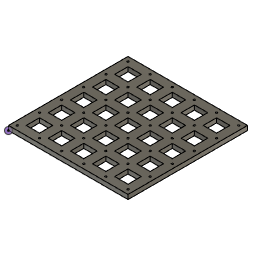
Base1 (Autodesk Fusion 360 design; units mm, degrees)
Autodesk Fusion 360 part; units mm, degrees
sketch "Sketch1" plane through (0, 0, 0) normal (0, 0, 1) x (1, 0, 0) in component "Base"
sketch "Sketch2" plane through (0, 0, 0) normal (0, 0, 1) x (1, 0, 0) in component "Base"
  line L0 (0, 0) -> (135, 0)
  line L1 (135, 0) -> (135, 135)
  line L2 (135, 135) -> (0, 135)
  line L3 (0, 135) -> (0, 0)
  line L4 (10, 10) -> (25, 10)
  line L5 (25, 10) -> (25, 25)
  line L6 (25, 25) -> (10, 25)
  line L7 (10, 25) -> (10, 10)
  line L8 (10, 35) -> (10, 50)
  line L9 (10, 50) -> (25, 50)
  line L10 (25, 50) -> (25, 35)
  line L11 (25, 35) -> (10, 35)
  line L12 (10, 60) -> (10, 75)
  line L13 (10, 75) -> (25, 75)
  line L14 (25, 75) -> (25, 60)
  line L15 (25, 60) -> (10, 60)
  line L16 (10, 85) -> (10, 100)
  line L17 (10, 100) -> (25, 100)
  line L18 (25, 100) -> (25, 85)
  line L19 (25, 85) -> (10, 85)
  line L20 (10, 110) -> (10, 125)
  line L21 (10, 125) -> (25, 125)
  line L22 (25, 125) -> (25, 110)
  line L23 (25, 110) -> (10, 110)
  line L24 (35, 125) -> (50, 125)
  line L25 (50, 125) -> (50, 110)
  line L26 (50, 110) -> (35, 110)
  line L27 (35, 110) -> (35, 125)
  line L28 (60, 110) -> (75, 110)
  line L29 (75, 110) -> (75, 125)
  line L30 (75, 125) -> (60, 125)
  line L31 (60, 125) -> (60, 110)
  line L32 (85, 110) -> (100, 110)
  line L33 (100, 110) -> (100, 125)
  line L34 (100, 125) -> (85, 125)
  line L35 (85, 125) -> (85, 110)
  line L36 (110, 110) -> (125, 110)
  line L37 (125, 110) -> (125, 125)
  line L38 (125, 125) -> (110, 125)
  line L39 (110, 125) -> (110, 110)
  line L40 (125, 100) -> (110, 100)
  line L41 (110, 100) -> (110, 85)
  line L42 (110, 85) -> (125, 85)
  line L43 (125, 85) -> (125, 100)
  line L44 (125, 75) -> (110, 75)
  line L45 (110, 75) -> (110, 60)
  line L46 (110, 60) -> (125, 60)
  line L47 (125, 60) -> (125, 75)
  line L48 (125, 50) -> (110, 50)
  line L49 (110, 50) -> (110, 35)
  line L50 (110, 35) -> (125, 35)
  line L51 (125, 35) -> (125, 50)
  line L52 (125, 25) -> (110, 25)
  line L53 (110, 25) -> (110, 10)
  line L54 (110, 10) -> (125, 10)
  line L55 (125, 10) -> (125, 25)
  line L56 (100, 10) -> (85, 10)
  line L57 (85, 10) -> (85, 25)
  line L58 (85, 25) -> (100, 25)
  line L59 (100, 25) -> (100, 10)
  line L60 (75, 10) -> (60, 10)
  line L61 (60, 10) -> (60, 25)
  line L62 (60, 25) -> (75, 25)
  line L63 (75, 25) -> (75, 10)
  line L64 (50, 10) -> (35, 10)
  line L65 (35, 10) -> (35, 25)
  line L66 (35, 25) -> (50, 25)
  line L67 (50, 25) -> (50, 10)
  line L68 (35, 35) -> (50, 35)
  line L69 (50, 35) -> (50, 50)
  line L70 (50, 50) -> (35, 50)
  line L71 (35, 50) -> (35, 35)
  line L72 (35, 60) -> (50, 60)
  line L73 (50, 60) -> (50, 75)
  line L74 (50, 75) -> (35, 75)
  line L75 (35, 75) -> (35, 60)
  line L76 (35, 85) -> (50, 85)
  line L77 (50, 85) -> (50, 100)
  line L78 (50, 100) -> (35, 100)
  line L79 (35, 100) -> (35, 85)
  line L80 (60, 100) -> (75, 100)
  line L81 (75, 100) -> (75, 85)
  line L82 (75, 85) -> (60, 85)
  line L83 (60, 85) -> (60, 100)
  line L84 (85, 100) -> (100, 100)
  line L85 (100, 100) -> (100, 85)
  line L86 (100, 85) -> (85, 85)
  line L87 (85, 85) -> (85, 100)
  line L88 (85, 75) -> (100, 75)
  line L89 (100, 75) -> (100, 60)
  line L90 (100, 60) -> (85, 60)
  line L91 (85, 60) -> (85, 75)
  line L92 (85, 50) -> (100, 50)
  line L93 (100, 50) -> (100, 35)
  line L94 (100, 35) -> (85, 35)
  line L95 (85, 35) -> (85, 50)
  line L96 (75, 35) -> (60, 35)
  line L97 (60, 35) -> (60, 50)
  line L98 (60, 50) -> (75, 50)
  line L99 (75, 50) -> (75, 35)
  line L100 (60, 60) -> (75, 60)
  line L101 (75, 60) -> (75, 75)
  line L102 (75, 75) -> (60, 75)
  line L103 (60, 75) -> (60, 60)
  circle A0 centre (5, 130) radius 1
  circle A1 centre (30, 130) radius 1
  circle A2 centre (55, 130) radius 1
  circle A3 centre (80, 130) radius 1
  circle A4 centre (105, 130) radius 1
  circle A5 centre (130, 130) radius 1
  circle A6 centre (105, 105) radius 1
  circle A7 centre (130, 105) radius 1
  circle A8 centre (5, 105) radius 1
  circle A9 centre (55, 105) radius 1
  circle A10 centre (80, 105) radius 1
  circle A11 centre (30, 105) radius 1
  circle A12 centre (105, 80) radius 1
  circle A13 centre (130, 80) radius 1
  circle A14 centre (5, 80) radius 1
  circle A15 centre (55, 80) radius 1
  circle A16 centre (80, 80) radius 1
  circle A17 centre (30, 80) radius 1
  circle A18 centre (105, 55) radius 1
  circle A19 centre (130, 55) radius 1
  circle A20 centre (5, 55) radius 1
  circle A21 centre (55, 55) radius 1
  circle A22 centre (80, 55) radius 1
  circle A23 centre (30, 55) radius 1
  circle A24 centre (105, 30) radius 1
  circle A25 centre (130, 30) radius 1
  circle A26 centre (5, 30) radius 1
  circle A27 centre (55, 30) radius 1
  circle A28 centre (80, 30) radius 1
  circle A29 centre (30, 30) radius 1
  circle A30 centre (105, 5) radius 1
  circle A31 centre (130, 5) radius 1
  circle A32 centre (5, 5) radius 1
  circle A33 centre (55, 5) radius 1
  circle A34 centre (80, 5) radius 1
  circle A35 centre (30, 5) radius 1
  point P0 (10, 10)
  point P1 (125, 10)
  point P2 (125, 125)
  point P3 (10, 125)
  point P4 (10, 110)
  point P5 (10, 100)
  point P6 (10, 85)
  point P7 (10, 75)
  point P8 (10, 60)
  point P9 (10, 50)
  point P10 (10, 35)
  point P11 (10, 25)
  point P12 (25, 10)
  point P13 (35, 10)
  point P14 (50, 10)
  point P15 (60, 10)
  point P16 (75, 10)
  point P17 (85, 10)
  point P18 (100, 10)
  point P19 (110, 10)
  point P20 (125, 25)
  point P21 (125, 35)
  point P22 (125, 50)
  point P23 (125, 60)
  point P24 (125, 75)
  point P25 (125, 85)
  point P26 (125, 100)
  point P27 (125, 110)
  point P28 (110, 125)
  point P29 (100, 125)
  point P30 (85, 125)
  point P31 (75, 125)
  point P32 (60, 125)
  point P33 (50, 125)
  point P34 (35, 125)
  point P35 (25, 125)
  point P36 (25, 110)
  point P37 (25, 100)
  point P38 (25, 85)
  point P39 (25, 75)
  point P40 (25, 60)
  point P41 (25, 50)
  point P42 (25, 35)
  point P43 (25, 25)
  point P44 (35, 25)
  point P45 (50, 25)
  point P46 (60, 25)
  point P47 (75, 25)
  point P48 (85, 25)
  point P49 (100, 25)
  point P50 (110, 25)
  point P51 (110, 35)
  point P52 (110, 50)
  point P53 (110, 60)
  point P54 (110, 75)
  point P55 (110, 85)
  point P56 (110, 100)
  point P57 (110, 110)
  point P58 (100, 110)
  point P59 (85, 110)
  point P60 (75, 110)
  point P61 (60, 110)
  point P62 (50, 110)
  point P63 (35, 110)
  point P64 (35, 100)
  point P65 (35, 85)
  point P66 (35, 75)
  point P67 (35, 60)
  point P68 (35, 50)
  point P69 (35, 35)
  point P70 (50, 35)
  point P71 (60, 35)
  point P72 (75, 35)
  point P73 (85, 35)
  point P74 (100, 35)
  point P75 (100, 50)
  point P76 (100, 60)
  point P77 (100, 75)
  point P78 (100, 85)
  point P79 (100, 100)
  point P80 (85, 100)
  point P81 (75, 100)
  point P82 (60, 100)
  point P83 (50, 100)
  point P84 (50, 85)
  point P85 (50, 75)
  point P86 (50, 60)
  point P87 (50, 50)
  point P88 (60, 50)
  point P89 (75, 50)
  point P90 (85, 50)
  point P91 (85, 60)
  point P92 (85, 75)
  point P93 (85, 85)
  point P94 (75, 85)
  point P95 (60, 85)
  point P96 (60, 75)
  point P97 (60, 60)
  point P98 (75, 60)
  point P99 (75, 75)
  dimension "d8" = 135
  dimension "d9" = 135
  dimension "d12" = 2
  dimension "d13" = 2
  dimension "d14" = 2
  dimension "d15" = 2
  dimension "d16" = 2
  dimension "d17" = 2
  dimension "d24" = 2
  dimension "d25" = 2
  dimension "d26" = 2
  dimension "d27" = 2
  dimension "d28" = 2
  dimension "d29" = 2
  dimension "d30" = 2
  dimension "d31" = 2
  dimension "d32" = 2
  dimension "d33" = 2
  dimension "d34" = 2
  dimension "d35" = 2
  dimension "d36" = 2
  dimension "d37" = 2
  dimension "d38" = 2
  dimension "d39" = 2
  dimension "d40" = 2
  dimension "d41" = 2
  dimension "d42" = 2
  dimension "d43" = 2
  dimension "d44" = 2
  dimension "d45" = 2
  dimension "d46" = 2
  dimension "d47" = 2
  dimension "d48" = 2
  dimension "d49" = 2
  dimension "d50" = 2
  dimension "d51" = 2
  dimension "d52" = 2
  dimension "d53" = 2
  constraint horizontal L0
  constraint vertical L1
  constraint horizontal L2
  constraint vertical L3
  constraint coincident L0.start L3.end
  constraint coincident P0 L4.start
  constraint coincident P12 L4.end
  constraint perpendicular L3 L4
  constraint coincident P43 L5.end
  constraint perpendicular L4 L5
  constraint coincident P11 L6.end
  constraint perpendicular L5 L6
  constraint perpendicular L4 L7
  constraint coincident P10 L8.start
  constraint coincident P9 L8.end
  constraint parallel L3 L8
  constraint coincident P41 L9.end
  constraint perpendicular L3 L9
  constraint coincident P42 L10.end
  constraint perpendicular L9 L10
  constraint perpendicular L8 L11
  constraint coincident P8 L12.start
  constraint coincident P7 L12.end
  constraint vertical L12
  constraint coincident P39 L13.end
  constraint perpendicular L12 L13
  constraint coincident P40 L14.end
  constraint perpendicular L13 L14
  constraint perpendicular L12 L15
  constraint coincident P6 L16.start
  constraint coincident P5 L16.end
  constraint vertical L16
  constraint coincident P37 L17.end
  constraint perpendicular L16 L17
  constraint coincident P38 L18.end
  constraint perpendicular L17 L18
  constraint perpendicular L16 L19
  constraint coincident P4 L20.start
  constraint coincident P3 L20.end
  constraint vertical L20
  constraint coincident P35 L21.end
  constraint perpendicular L20 L21
  constraint coincident P36 L22.end
  constraint perpendicular L21 L22
  constraint perpendicular L20 L23
  constraint coincident P34 L24.start
  constraint coincident P33 L24.end
  constraint horizontal L24
  constraint coincident P62 L25.end
  constraint perpendicular L24 L25
  constraint coincident P63 L26.end
  constraint perpendicular L25 L26
  constraint perpendicular L24 L27
  constraint horizontal L28
  constraint vertical L29
  constraint horizontal L30
  constraint vertical L31
  constraint coincident P31 L29.end
  constraint coincident P61 L28.start
  constraint horizontal L32
  constraint vertical L33
  constraint horizontal L34
  constraint vertical L35
  constraint coincident P29 L33.end
  constraint coincident P59 L32.start
  constraint horizontal L36
  constraint vertical L37
  constraint horizontal L38
  constraint vertical L39
  constraint coincident P2 L37.end
  constraint coincident P57 L36.start
  constraint horizontal L40
  constraint vertical L41
  constraint horizontal L42
  constraint vertical L43
  constraint coincident P55 L41.end
  constraint coincident P26 L40.start
  constraint horizontal L44
  constraint vertical L45
  constraint horizontal L46
  constraint vertical L47
  constraint coincident P53 L45.end
  constraint coincident P24 L44.start
  constraint horizontal L48
  constraint vertical L49
  constraint horizontal L50
  constraint vertical L51
  constraint coincident P51 L49.end
  constraint coincident P22 L48.start
  constraint horizontal L52
  constraint vertical L53
  constraint horizontal L54
  constraint vertical L55
  constraint coincident P19 L53.end
  constraint coincident P20 L52.start
  constraint horizontal L56
  constraint vertical L57
  constraint horizontal L58
  constraint vertical L59
  constraint coincident P48 L57.end
  constraint coincident P18 L56.start
  constraint horizontal L60
  constraint vertical L61
  constraint horizontal L62
  constraint vertical L63
  constraint coincident P46 L61.end
  constraint coincident P16 L60.start
  constraint horizontal L64
  constraint vertical L65
  constraint horizontal L66
  constraint vertical L67
  constraint coincident P44 L65.end
  constraint coincident P14 L64.start
  constraint horizontal L68
  constraint vertical L69
  constraint horizontal L70
  constraint vertical L71
  constraint coincident P87 L69.end
  constraint coincident P69 L68.start
  constraint horizontal L72
  constraint vertical L73
  constraint horizontal L74
  constraint vertical L75
  constraint coincident P85 L73.end
  constraint coincident P67 L72.start
  constraint horizontal L76
  constraint vertical L77
  constraint horizontal L78
  constraint vertical L79
  constraint coincident P83 L77.end
  constraint coincident P65 L76.start
  constraint horizontal L80
  constraint vertical L81
  constraint horizontal L82
  constraint vertical L83
  constraint coincident P94 L81.end
  constraint coincident P82 L80.start
  constraint horizontal L84
  constraint vertical L85
  constraint horizontal L86
  constraint vertical L87
  constraint coincident P78 L85.end
  constraint coincident P80 L84.start
  constraint horizontal L88
  constraint vertical L89
  constraint horizontal L90
  constraint vertical L91
  constraint coincident P76 L89.end
  constraint coincident P92 L88.start
  constraint horizontal L92
  constraint vertical L93
  constraint horizontal L94
  constraint vertical L95
  constraint coincident P74 L93.end
  constraint coincident P90 L92.start
  constraint horizontal L96
  constraint vertical L97
  constraint horizontal L98
  constraint vertical L99
  constraint coincident P88 L97.end
  constraint coincident P72 L96.start
  constraint horizontal L100
  constraint vertical L101
  constraint horizontal L102
  constraint vertical L103
  constraint coincident P99 L101.end
  constraint coincident P97 L100.start
  measures "d8" distance of L0.start L0.end
  measures "d9" distance of L0.start L2.end
  measures "d12" diameter of A0
  measures "d13" diameter of A1
  measures "d14" diameter of A2
  measures "d15" diameter of A3
  measures "d16" diameter of A4
  measures "d17" diameter of A5
  measures "d24" diameter of A8
  measures "d25" diameter of A11
  measures "d26" diameter of A9
  measures "d27" diameter of A10
  measures "d28" diameter of A6
  measures "d29" diameter of A7
  measures "d30" diameter of A14
  measures "d31" diameter of A17
  measures "d32" diameter of A15
  measures "d33" diameter of A16
  measures "d34" diameter of A12
  measures "d35" diameter of A13
  measures "d36" diameter of A20
  measures "d37" diameter of A23
  measures "d38" diameter of A21
  measures "d39" diameter of A22
  measures "d40" diameter of A18
  measures "d41" diameter of A19
  measures "d42" diameter of A26
  measures "d43" diameter of A29
  measures "d44" diameter of A27
  measures "d45" diameter of A28
  measures "d46" diameter of A24
  measures "d47" diameter of A25
  measures "d48" diameter of A32
  measures "d49" diameter of A35
  measures "d50" diameter of A33
  measures "d51" diameter of A34
  measures "d52" diameter of A30
  measures "d53" diameter of A31
extrude "Extrude1" add sketch "Sketch2" along normal blind 5 in component "Base"
component "Base" placed x (1, 0, 0) y (0, 1, 0) z (0, 0, 1) at (0, 0, 0)
